Autodesk Fusion 360 part; units mm, degrees
(part 4 of 5)
sketch "Sketch4" plane through (0, 0, 22) normal (0, 0, 1) x (-1, 0, 0)
  spline S0 degree 3 poles (-268.4797, 103.3781) (-268.5106, 103.349) (-268.5781, 103.2853) (-268.6125, 103.1987) (-268.6312, 103.1517) knots 0 0 0 0 0.012573 0.027537 0.027537 0.027537 0.027537
  line L0 (-268.6312, 103.1517) -> (-268.8849, 103.183)
  spline S1 degree 3 poles (-269.284, 103.5337) (-269.2388, 103.4878) (-269.1427, 103.3903) (-269.1115, 103.2566) (-269.095, 103.1858) knots 0 0 0 0 0.01895 0.040278 0.040278 0.040278 0.040278
  line L1 (-269.095, 103.1858) -> (-269.3379, 103.1476)
  spline S2 degree 3 poles (-269.713, 103.4491) (-269.7635, 103.4479) (-269.8534, 103.4458) (-269.9303, 103.4002) (-269.9641, 103.3802) knots 0 0 0 0 0.014834 0.026419 0.026419 0.026419 0.026419
  spline S3 degree 3 poles (-269.9641, 103.3802) (-269.9879, 103.3569) (-270.0338, 103.3122) (-270.042, 103.2489) (-270.0459, 103.2185) knots 0 0 0 0 0.009682 0.0186 0.0186 0.0186 0.0186
  spline S4 degree 3 poles (-269.4572, 102.166) (-269.4912, 102.1574) (-269.5609, 102.1399) (-269.6326, 102.1378) (-269.6694, 102.1367) knots 0 0 0 0 0.010482 0.021472 0.021472 0.021472 0.021472
  spline S5 degree 3 poles (-269.6694, 102.1367) (-269.7232, 102.1382) (-269.8253, 102.1412) (-269.9227, 102.1715) (-269.9688, 102.1858) knots 0 0 0 0 0.01606 0.030471 0.030471 0.030471 0.030471
  spline S6 degree 3 poles (-252.8144, 103.5848) (-252.7657, 103.5945) (-252.6592, 103.6158) (-252.5506, 103.6174) (-252.4917, 103.6182) knots 0 0 0 0 0.014862 0.032497 0.032497 0.032497 0.032497
  line L2 (-252.4917, 103.6182) -> (-251.7291, 103.6182)
  line L3 (-251.7291, 103.6182) -> (-251.7291, 101.6182)
  line L4 (-251.7291, 101.6182) -> (-252.4794, 101.6182)
  spline S7 degree 3 poles (-252.4794, 101.6182) (-252.5489, 101.6195) (-252.6746, 101.6218) (-252.7938, 101.6613) (-252.8471, 101.6789) knots 0 0 0 0 0.020707 0.037453 0.037453 0.037453 0.037453
  spline S8 degree 3 poles (-252.8471, 101.6789) (-252.8907, 101.7018) (-252.9775, 101.7473) (-253.0353, 101.8265) (-253.064, 101.8658) knots 0 0 0 0 0.014555 0.028975 0.028975 0.028975 0.028975
  spline S9 degree 3 poles (-253.064, 101.8658) (-253.0869, 101.9079) (-253.1317, 101.9904) (-253.1389, 102.084) (-253.1425, 102.1298) knots 0 0 0 0 0.014187 0.027818 0.027818 0.027818 0.027818
  spline S10 degree 3 poles (-253.1425, 102.1298) (-253.1394, 102.1721) (-253.1334, 102.2575) (-253.0932, 102.3331) (-253.0729, 102.3713) knots 0 0 0 0 0.01257 0.025379 0.025379 0.025379 0.025379
  spline S11 degree 3 poles (-253.0729, 102.3713) (-253.0458, 102.4077) (-252.9891, 102.4838) (-252.9061, 102.53) (-252.8628, 102.5541) knots 0 0 0 0 0.013451 0.028132 0.028132 0.028132 0.028132
  spline S12 degree 3 poles (-252.8628, 102.5541) (-252.919, 102.574) (-253.0268, 102.6121) (-253.1046, 102.6956) (-253.1418, 102.7356) knots 0 0 0 0 0.017587 0.033722 0.033722 0.033722 0.033722
  spline S13 degree 3 poles (-253.1418, 102.7356) (-253.1702, 102.7808) (-253.2284, 102.8734) (-253.2356, 102.9826) (-253.2393, 103.0384) knots 0 0 0 0 0.015782 0.032266 0.032266 0.032266 0.032266
  spline S14 degree 3 poles (-253.2393, 103.0384) (-253.237, 103.0842) (-253.2323, 103.1747) (-253.1973, 103.2584) (-253.18, 103.2997) knots 0 0 0 0 0.013638 0.026971 0.026971 0.026971 0.026971
  spline S15 degree 3 poles (-253.18, 103.2997) (-253.1599, 103.3369) (-253.1218, 103.4076) (-253.0617, 103.4608) (-253.0333, 103.4859) knots 0 0 0 0 0.012583 0.02387 0.02387 0.02387 0.02387
  spline S16 degree 3 poles (-253.0333, 103.4859) (-253.0013, 103.5067) (-252.9333, 103.5507) (-252.8555, 103.573) (-252.8144, 103.5848) knots 0 0 0 0 0.011395 0.024144 0.024144 0.024144 0.024144
  spline S17 degree 3 poles (-257.0244, 103.3904) (-257.0362, 103.3956) (-257.0628, 103.4073) (-257.092, 103.4078) (-257.1083, 103.4081) knots 0 0 0 0 0.003804 0.008651 0.008651 0.008651 0.008651
  spline S18 degree 3 poles (-257.1083, 103.4081) (-257.1242, 103.4076) (-257.1603, 103.4063) (-257.196, 103.4014) (-257.2161, 103.3986) knots 0 0 0 0 0.004747 0.010826 0.010826 0.010826 0.010826
  line L5 (-257.2161, 103.3986) -> (-257.2516, 103.6155)
  spline S19 degree 3 poles (-257.2516, 103.6155) (-257.219, 103.6219) (-257.1576, 103.6338) (-257.0952, 103.6362) (-257.0661, 103.6373) knots 0 0 0 0 0.009958 0.018706 0.018706 0.018706 0.018706
  spline S20 degree 3 poles (-257.0661, 103.6373) (-257.0259, 103.6366) (-256.954, 103.6352) (-256.8879, 103.6073) (-256.8587, 103.595) knots 0 0 0 0 0.011916 0.021334 0.021334 0.021334 0.021334
  spline S21 degree 3 poles (-256.8587, 103.595) (-256.8361, 103.5802) (-256.7925, 103.5516) (-256.7672, 103.5059) (-256.755, 103.4839) knots 0 0 0 0 0.007958 0.015408 0.015408 0.015408 0.015408
  spline S22 degree 3 poles (-256.755, 103.4839) (-256.7464, 103.4484) (-256.7233, 103.3534) (-256.7243, 103.2553) (-256.725, 103.194) knots 0 0 0 0 0.010927 0.02924 0.02924 0.02924 0.02924
  line L6 (-256.725, 103.194) -> (-256.725, 102.3604)
  line L7 (-256.725, 102.3604) -> (-256.5449, 102.3604)
  line L8 (-256.5449, 102.3604) -> (-256.5449, 102.1694)
  line L9 (-256.5449, 102.1694) -> (-256.725, 102.1694)
  line L10 (-256.725, 102.1694) -> (-256.725, 101.8106)
  line L11 (-256.725, 101.8106) -> (-256.9692, 101.6633)
  line L12 (-256.9692, 101.6633) -> (-256.9692, 102.1694)
  line L13 (-256.9692, 102.1694) -> (-257.2161, 102.1694)
  line L14 (-257.2161, 102.1694) -> (-257.2161, 102.3604)
  line L15 (-257.2161, 102.3604) -> (-256.9692, 102.3604)
  line L16 (-256.9692, 102.3604) -> (-256.9692, 103.2076)
  spline S23 degree 3 poles (-256.9692, 103.2076) (-256.9688, 103.2365) (-256.9683, 103.2821) (-256.9784, 103.3265) (-256.9822, 103.3427) knots 0 0 0 0 0.008635 0.013608 0.013608 0.013608 0.013608
  spline S24 degree 3 poles (-256.9822, 103.3427) (-256.9872, 103.3522) (-256.9975, 103.3715) (-257.0154, 103.384) (-257.0244, 103.3904) knots 0 0 0 0 0.003189 0.00646 0.00646 0.00646 0.00646
  line L17 (-278.1333, 51.124) -> (-278.1333, 51.9371)
  line L18 (-278.1333, 51.9371) -> (-277.8686, 51.9371)
  line L19 (-277.8686, 51.9371) -> (-277.8686, 49.9371)
  line L20 (-277.8686, 49.9371) -> (-278.623, 49.9371)
  spline S25 degree 3 poles (-278.623, 49.9371) (-278.6817, 49.9373) (-278.7835, 49.9376) (-278.8844, 49.9507) (-278.9272, 49.9562) knots 0 0 0 0 0.017571 0.030509 0.030509 0.030509 0.030509
  spline S26 degree 3 poles (-278.9272, 49.9562) (-278.9734, 49.9656) (-279.0608, 49.9833) (-279.1378, 50.0284) (-279.1742, 50.0497) knots 0 0 0 0 0.014001 0.026564 0.026564 0.026564 0.026564
  spline S27 degree 3 poles (-279.1742, 50.0497) (-279.2061, 50.0756) (-279.2722, 50.1294) (-279.3132, 50.2041) (-279.3345, 50.2427) knots 0 0 0 0 0.012214 0.025303 0.025303 0.025303 0.025303
  spline S28 degree 3 poles (-279.3345, 50.2427) (-279.3522, 50.2856) (-279.3883, 50.373) (-279.3929, 50.4675) (-279.3952, 50.5156) knots 0 0 0 0 0.013801 0.028138 0.028138 0.028138 0.028138
  spline S29 degree 3 poles (-279.3952, 50.5156) (-279.3889, 50.5968) (-279.3765, 50.7566) (-279.2802, 50.8845) (-279.2328, 50.9474) knots 0 0 0 0 0.023898 0.046996 0.046996 0.046996 0.046996
  spline S30 degree 3 poles (-279.2328, 50.9474) (-279.1593, 50.9986) (-278.9848, 51.1201) (-278.7703, 51.1226) (-278.6462, 51.124) knots 0 0 0 0 0.026356 0.062507 0.062507 0.062507 0.062507
  line L21 (-278.6462, 51.124) -> (-278.1333, 51.124)
  line L22 (-285.0691, 51.1786) -> (-285.0691, 51.9371)
  line L23 (-285.0691, 51.9371) -> (-284.8236, 51.9371)
  line L24 (-284.8236, 51.9371) -> (-284.8236, 50.4883)
  line L25 (-284.8236, 50.4883) -> (-285.0446, 50.4883)
  line L26 (-285.0446, 50.4883) -> (-285.0446, 50.7079)
  spline S31 degree 3 poles (-285.0446, 50.7079) (-285.0692, 50.6633) (-285.1111, 50.5874) (-285.1746, 50.5288) (-285.2008, 50.5047) knots 0 0 0 0 0.015158 0.025781 0.025781 0.025781 0.025781
  spline S32 degree 3 poles (-285.2008, 50.5047) (-285.2252, 50.4904) (-285.2739, 50.4618) (-285.3303, 50.4576) (-285.3584, 50.4556) knots 0 0 0 0 0.008374 0.016702 0.016702 0.016702 0.016702
  spline S33 degree 3 poles (-285.3584, 50.4556) (-285.4009, 50.4595) (-285.4906, 50.4677) (-285.5693, 50.5116) (-285.6107, 50.5347) knots 0 0 0 0 0.012672 0.02671 0.02671 0.02671 0.02671
  line L27 (-285.6107, 50.5347) -> (-285.5262, 50.7625)
  spline S34 degree 3 poles (-285.5262, 50.7625) (-285.4968, 50.747) (-285.4403, 50.7172) (-285.3766, 50.7119) (-285.3461, 50.7093) knots 0 0 0 0 0.009849 0.018951 0.018951 0.018951 0.018951
  spline S35 degree 3 poles (-285.3461, 50.7093) (-285.3199, 50.7113) (-285.2677, 50.7154) (-285.2235, 50.7436) (-285.2015, 50.7577) knots 0 0 0 0 0.007735 0.015463 0.015463 0.015463 0.015463
  spline S36 degree 3 poles (-285.2015, 50.7577) (-285.1815, 50.7759) (-285.1403, 50.8133) (-285.1203, 50.8653) (-285.1101, 50.8921) knots 0 0 0 0 0.007973 0.016455 0.016455 0.016455 0.016455
  spline S37 degree 3 poles (-285.1101, 50.8921) (-285.0981, 50.9376) (-285.0735, 51.0315) (-285.0706, 51.1285) (-285.0691, 51.1786) knots 0 0 0 0 0.01405 0.029024 0.029024 0.029024 0.029024
  spline S38 degree 3 poles (-283.8822, 51.768) (-283.925, 51.7654) (-284.0078, 51.7606) (-284.0786, 51.7177) (-284.1128, 51.697) knots 0 0 0 0 0.012642 0.024448 0.024448 0.024448 0.024448
  spline S39 degree 3 poles (-284.1128, 51.697) (-284.1436, 51.6679) (-284.2112, 51.6042) (-284.2455, 51.5176) (-284.2642, 51.4706) knots 0 0 0 0 0.012573 0.027537 0.027537 0.027537 0.027537
  line L28 (-284.2642, 51.4706) -> (-284.518, 51.5019)
  spline S40 degree 3 poles (-284.518, 51.5019) (-284.4947, 51.5712) (-284.4495, 51.7052) (-284.3458, 51.8009) (-284.2956, 51.8471) knots 0 0 0 0 0.021523 0.041652 0.041652 0.041652 0.041652
  spline S41 degree 3 poles (-284.2956, 51.8471) (-284.2355, 51.8829) (-284.108, 51.9588) (-283.9595, 51.9661) (-283.8809, 51.9699) knots 0 0 0 0 0.020652 0.043844 0.043844 0.043844 0.043844
  spline S42 degree 3 poles (-283.8809, 51.9699) (-283.782, 51.9633) (-283.5929, 51.9508) (-283.4466, 51.8312) (-283.3768, 51.7741) knots 0 0 0 0 0.028913 0.055291 0.055291 0.055291 0.055291
  spline S43 degree 3 poles (-283.3768, 51.7741) (-283.3225, 51.6985) (-283.2054, 51.535) (-283.1957, 51.3333) (-283.1906, 51.225) knots 0 0 0 0 0.027351 0.059089 0.059089 0.059089 0.059089
  spline S44 degree 3 poles (-283.1906, 51.225) (-283.1957, 51.1131) (-283.2051, 50.9053) (-283.324, 50.7357) (-283.3788, 50.6575) knots 0 0 0 0 0.032809 0.060899 0.060899 0.060899 0.060899
  spline S45 degree 3 poles (-283.3788, 50.6575) (-283.4474, 50.5986) (-283.5878, 50.478) (-283.7726, 50.4631) (-283.8672, 50.4556) knots 0 0 0 0 0.026399 0.05408 0.05408 0.05408 0.05408
  spline S46 degree 3 poles (-283.8672, 50.4556) (-283.959, 50.4631) (-284.1388, 50.4779) (-284.2752, 50.5957) (-284.342, 50.6534) knots 0 0 0 0 0.026858 0.052633 0.052633 0.052633 0.052633
  spline S47 degree 3 poles (-284.342, 50.6534) (-284.3956, 50.7301) (-284.512, 50.8965) (-284.5212, 51.1002) (-284.5262, 51.21) knots 0 0 0 0 0.027523 0.05971 0.05971 0.05971 0.05971
  spline S48 degree 3 poles (-284.5262, 51.21) (-284.5261, 51.2191) (-284.5259, 51.2409) (-284.5252, 51.2627) (-284.5248, 51.2755) knots 0 0 0 0 0.002729 0.00655 0.00655 0.00655 0.00655
  line L29 (-284.5248, 51.2755) -> (-283.4443, 51.2755)
  spline S49 degree 3 poles (-283.4443, 51.2755) (-283.4514, 51.3482) (-283.4645, 51.4824) (-283.5433, 51.5913) (-283.5794, 51.6411) knots 0 0 0 0 0.021465 0.039604 0.039604 0.039604 0.039604
  spline S50 degree 3 poles (-283.5794, 51.6411) (-283.6226, 51.6781) (-283.7099, 51.7528) (-283.8244, 51.7629) (-283.8822, 51.768) knots 0 0 0 0 0.016633 0.033577 0.033577 0.033577 0.033577
  spline S51 degree 3 poles (-268.9524, 51.4636) (-268.9641, 51.4687) (-268.9908, 51.4805) (-269.02, 51.481) (-269.0363, 51.4813) knots 0 0 0 0 0.003804 0.008651 0.008651 0.008651 0.008651
  spline S52 degree 3 poles (-269.0363, 51.4813) (-269.0522, 51.4808) (-269.0882, 51.4795) (-269.124, 51.4745) (-269.1441, 51.4718) knots 0 0 0 0 0.004747 0.010826 0.010826 0.010826 0.010826
  line L30 (-269.1441, 51.4718) -> (-269.1796, 51.6887)
  spline S53 degree 3 poles (-269.1796, 51.6887) (-269.1469, 51.6951) (-269.0856, 51.707) (-269.0232, 51.7094) (-268.994, 51.7105) knots 0 0 0 0 0.009958 0.018706 0.018706 0.018706 0.018706
  spline S54 degree 3 poles (-268.994, 51.7105) (-268.9539, 51.7098) (-268.882, 51.7084) (-268.8159, 51.6805) (-268.7867, 51.6682) knots 0 0 0 0 0.011916 0.021334 0.021334 0.021334 0.021334
  spline S55 degree 3 poles (-268.7867, 51.6682) (-268.7641, 51.6534) (-268.7204, 51.6248) (-268.6952, 51.5791) (-268.683, 51.557) knots 0 0 0 0 0.007958 0.015408 0.015408 0.015408 0.015408
  spline S56 degree 3 poles (-268.683, 51.557) (-268.6744, 51.5215) (-268.6513, 51.4265) (-268.6523, 51.3285) (-268.653, 51.2671) knots 0 0 0 0 0.010927 0.02924 0.02924 0.02924 0.02924
  line L31 (-268.653, 51.2671) -> (-268.653, 50.4336)
  line L32 (-268.653, 50.4336) -> (-268.4729, 50.4336)
  line L33 (-268.4729, 50.4336) -> (-268.4729, 50.2426)
  line L34 (-268.4729, 50.2426) -> (-268.653, 50.2426)
  line L35 (-268.653, 50.2426) -> (-268.653, 49.8838)
  line L36 (-268.653, 49.8838) -> (-268.8972, 49.7364)
  line L37 (-268.8972, 49.7364) -> (-268.8972, 50.2426)
  line L38 (-268.8972, 50.2426) -> (-269.1441, 50.2426)
  line L39 (-269.1441, 50.2426) -> (-269.1441, 50.4336)
  line L40 (-269.1441, 50.4336) -> (-268.8972, 50.4336)
  line L41 (-268.8972, 50.4336) -> (-268.8972, 51.2808)
  spline S57 degree 3 poles (-268.8972, 51.2808) (-268.8968, 51.3097) (-268.8962, 51.3553) (-268.9064, 51.3996) (-268.9101, 51.4158) knots 0 0 0 0 0.008635 0.013608 0.013608 0.013608 0.013608
  spline S58 degree 3 poles (-268.9101, 51.4158) (-268.9152, 51.4254) (-268.9255, 51.4447) (-268.9434, 51.4572) (-268.9524, 51.4636) knots 0 0 0 0 0.003189 0.00646 0.00646 0.00646 0.00646
  spline S59 degree 3 poles (-273.7894, 51.7242) (-273.7043, 51.7218) (-273.5507, 51.7174) (-273.4181, 51.641) (-273.359, 51.6068) knots 0 0 0 0 0.025053 0.045234 0.045234 0.045234 0.045234
  spline S60 degree 3 poles (-273.359, 51.6068) (-273.3138, 51.561) (-273.2177, 51.4635) (-273.1865, 51.3298) (-273.17, 51.259) knots 0 0 0 0 0.01895 0.040278 0.040278 0.040278 0.040278
  line L42 (-273.17, 51.259) -> (-273.4129, 51.2208)
  spline S61 degree 3 poles (-273.4129, 51.2208) (-273.4218, 51.2658) (-273.4388, 51.3513) (-273.4985, 51.4146) (-273.5268, 51.4445) knots 0 0 0 0 0.013461 0.025563 0.025563 0.025563 0.025563
  spline S62 degree 3 poles (-273.5268, 51.4445) (-273.5631, 51.4671) (-273.6428, 51.5167) (-273.7369, 51.5203) (-273.788, 51.5223) knots 0 0 0 0 0.012631 0.027679 0.027679 0.027679 0.027679
  spline S63 degree 3 poles (-273.788, 51.5223) (-273.8385, 51.5211) (-273.9284, 51.519) (-274.0053, 51.4734) (-274.0391, 51.4534) knots 0 0 0 0 0.014834 0.026419 0.026419 0.026419 0.026419
  spline S64 degree 3 poles (-274.0391, 51.4534) (-274.0629, 51.4301) (-274.1088, 51.3854) (-274.117, 51.3221) (-274.1209, 51.2917) knots 0 0 0 0 0.009682 0.0186 0.0186 0.0186 0.0186
  spline S65 degree 3 poles (-274.1209, 51.2917) (-274.1178, 51.2653) (-274.1114, 51.212) (-274.0697, 51.1779) (-274.0486, 51.1607) knots 0 0 0 0 0.007652 0.015492 0.015492 0.015492 0.015492
  spline S66 degree 3 poles (-274.0486, 51.1607) (-274.0195, 51.1477) (-273.9388, 51.1114) (-273.8527, 51.0907) (-273.7976, 51.0775) knots 0 0 0 0 0.009553 0.026493 0.026493 0.026493 0.026493
  spline S67 degree 3 poles (-273.7976, 51.0775) (-273.7207, 51.0583) (-273.5935, 51.0264) (-273.4714, 50.9785) (-273.4231, 50.9595) knots 0 0 0 0 0.023737 0.039299 0.039299 0.039299 0.039299
  spline S68 degree 3 poles (-273.4231, 50.9595) (-273.3907, 50.9418) (-273.3278, 50.9074) (-273.2854, 50.8497) (-273.2648, 50.8217) knots 0 0 0 0 0.010927 0.021211 0.021211 0.021211 0.021211
  spline S69 degree 3 poles (-273.2648, 50.8217) (-273.2491, 50.7915) (-273.2174, 50.7305) (-273.2131, 50.6619) (-273.211, 50.6273) knots 0 0 0 0 0.010103 0.020373 0.020373 0.020373 0.020373
  spline S70 degree 3 poles (-273.211, 50.6273) (-273.2127, 50.5957) (-273.2163, 50.5331) (-273.2424, 50.4762) (-273.2553, 50.4479) knots 0 0 0 0 0.009394 0.018625 0.018625 0.018625 0.018625
  spline S71 degree 3 poles (-273.2553, 50.4479) (-273.2714, 50.4216) (-273.3037, 50.3688) (-273.3519, 50.3301) (-273.376, 50.3108) knots 0 0 0 0 0.009191 0.018392 0.018392 0.018392 0.018392
  spline S72 degree 3 poles (-273.376, 50.3108) (-273.3982, 50.2969) (-273.447, 50.2661) (-273.5021, 50.2487) (-273.5322, 50.2392) knots 0 0 0 0 0.007816 0.017247 0.017247 0.017247 0.017247
  spline S73 degree 3 poles (-273.5322, 50.2392) (-273.5662, 50.2306) (-273.6359, 50.2131) (-273.7076, 50.2109) (-273.7444, 50.2098) knots 0 0 0 0 0.010482 0.021472 0.021472 0.021472 0.021472
  spline S74 degree 3 poles (-273.7444, 50.2098) (-273.7982, 50.2114) (-273.9003, 50.2144) (-273.9977, 50.2446) (-274.0438, 50.259) knots 0 0 0 0 0.01606 0.030471 0.030471 0.030471 0.030471
  spline S75 degree 3 poles (-274.0438, 50.259) (-274.0831, 50.2756) (-274.1561, 50.3065) (-274.2095, 50.3649) (-274.2342, 50.392) knots 0 0 0 0 0.012607 0.023462 0.023462 0.023462 0.023462
  spline S76 degree 3 poles (-274.2342, 50.392) (-274.2533, 50.4239) (-274.2949, 50.4935) (-274.3104, 50.5733) (-274.3187, 50.6164) knots 0 0 0 0 0.011092 0.024145 0.024145 0.024145 0.024145
  line L43 (-274.3187, 50.6164) -> (-274.0786, 50.6491)
  spline S77 degree 3 poles (-274.0786, 50.6491) (-274.071, 50.6143) (-274.0563, 50.5467) (-274.0075, 50.498) (-273.9838, 50.4745) knots 0 0 0 0 0.010457 0.02025 0.02025 0.02025 0.02025
  spline S78 degree 3 poles (-273.9838, 50.4745) (-273.953, 50.4562) (-273.885, 50.4159) (-273.8056, 50.4132) (-273.7621, 50.4118) knots 0 0 0 0 0.01057 0.023371 0.023371 0.023371 0.023371
  spline S79 degree 3 poles (-273.7621, 50.4118) (-273.7127, 50.4121) (-273.6276, 50.4128) (-273.5522, 50.4515) (-273.5206, 50.4677) knots 0 0 0 0 0.014563 0.025087 0.025087 0.025087 0.025087
  spline S80 degree 3 poles (-273.5206, 50.4677) (-273.4996, 50.4863) (-273.4597, 50.5216) (-273.452, 50.574) (-273.4483, 50.5987) knots 0 0 0 0 0.00814 0.015395 0.015395 0.015395 0.015395
  spline S81 degree 3 poles (-273.4483, 50.5987) (-273.4496, 50.6142) (-273.4522, 50.6454) (-273.4696, 50.6715) (-273.4784, 50.6846) knots 0 0 0 0 0.004598 0.009239 0.009239 0.009239 0.009239
  spline S82 degree 3 poles (-273.4784, 50.6846) (-273.4906, 50.6975) (-273.5173, 50.7258) (-273.5531, 50.7415) (-273.5725, 50.7501) knots 0 0 0 0 0.005284 0.01157 0.01157 0.01157 0.01157
  spline S83 degree 3 poles (-273.5725, 50.7501) (-273.5967, 50.7577) (-273.6685, 50.7803) (-273.7412, 50.7999) (-273.7894, 50.8128) knots 0 0 0 0 0.007605 0.022583 0.022583 0.022583 0.022583
  spline S84 degree 3 poles (-273.7894, 50.8128) (-273.8636, 50.8325) (-273.9865, 50.8652) (-274.1057, 50.9093) (-274.153, 50.9268) knots 0 0 0 0 0.023005 0.038118 0.038118 0.038118 0.038118
  spline S85 degree 3 poles (-274.153, 50.9268) (-274.1852, 50.9429) (-274.2483, 50.9744) (-274.2929, 51.029) (-274.3146, 51.0557) knots 0 0 0 0 0.010681 0.020888 0.020888 0.020888 0.020888
  spline S86 degree 3 poles (-274.3146, 51.0557) (-274.3317, 51.0866) (-274.3678, 51.1518) (-274.3714, 51.2265) (-274.3733, 51.2658) knots 0 0 0 0 0.010453 0.022074 0.022074 0.022074 0.022074
  spline S87 degree 3 poles (-274.3733, 51.2658) (-274.3701, 51.3064) (-274.3637, 51.3888) (-274.3226, 51.4606) (-274.3017, 51.497) knots 0 0 0 0 0.012054 0.024479 0.024479 0.024479 0.024479
  spline S88 degree 3 poles (-274.3017, 51.497) (-274.2745, 51.5314) (-274.2181, 51.6027) (-274.1369, 51.6436) (-274.095, 51.6648) knots 0 0 0 0 0.013001 0.026908 0.026908 0.026908 0.026908
  spline S89 degree 3 poles (-274.095, 51.6648) (-274.0475, 51.6821) (-273.9489, 51.7181) (-273.8439, 51.7221) (-273.7894, 51.7242) knots 0 0 0 0 0.015065 0.0313 0.0313 0.0313 0.0313
  line L44 (-272.8835, 50.2426) -> (-272.8835, 51.6914)
  line L45 (-272.8835, 51.6914) -> (-272.6639, 51.6914)
  line L46 (-272.6639, 51.6914) -> (-272.6639, 51.4786)
  spline S90 degree 3 poles (-272.6639, 51.4786) (-272.6028, 51.5502) (-272.4816, 51.6924) (-272.2962, 51.7136) (-272.2041, 51.7242) knots 0 0 0 0 0.027153 0.053891 0.053891 0.053891 0.053891
  spline S91 degree 3 poles (-272.2041, 51.7242) (-272.1624, 51.7222) (-272.08, 51.7184) (-272.0028, 51.6894) (-271.9647, 51.6751) knots 0 0 0 0 0.012458 0.024577 0.024577 0.024577 0.024577
  spline S92 degree 3 poles (-271.9647, 51.6751) (-271.9308, 51.6587) (-271.8677, 51.6281) (-271.8212, 51.5758) (-271.7996, 51.5516) knots 0 0 0 0 0.01116 0.020794 0.020794 0.020794 0.020794
  spline S93 degree 3 poles (-271.7996, 51.5516) (-271.7829, 51.5246) (-271.7477, 51.4681) (-271.7321, 51.4034) (-271.7239, 51.3695) knots 0 0 0 0 0.009458 0.019838 0.019838 0.019838 0.019838
  spline S94 degree 3 poles (-271.7239, 51.3695) (-271.7196, 51.3384) (-271.709, 51.2624) (-271.7089, 51.1856) (-271.7089, 51.1403) knots 0 0 0 0 0.009413 0.022992 0.022992 0.022992 0.022992
  line L47 (-271.7089, 51.1403) -> (-271.7089, 50.2426)
  line L48 (-271.7089, 50.2426) -> (-271.9545, 50.2426)
  line L49 (-271.9545, 50.2426) -> (-271.9545, 51.0461)
  spline S95 degree 3 poles (-271.9545, 51.0461) (-271.9542, 51.0999) (-271.9538, 51.1867) (-271.9652, 51.2726) (-271.9695, 51.3053) knots 0 0 0 0 0.016103 0.02599 0.02599 0.02599 0.02599
  spline S96 degree 3 poles (-271.9695, 51.3053) (-271.9791, 51.3357) (-271.9981, 51.3954) (-272.0448, 51.437) (-272.0677, 51.4575) knots 0 0 0 0 0.009371 0.018407 0.018407 0.018407 0.018407
  spline S97 degree 3 poles (-272.0677, 51.4575) (-272.095, 51.4736) (-272.1521, 51.5073) (-272.2185, 51.5109) (-272.2533, 51.5127) knots 0 0 0 0 0.009358 0.019615 0.019615 0.019615 0.019615
  spline S98 degree 3 poles (-272.2533, 51.5127) (-272.2896, 51.5103) (-272.3625, 51.5055) (-272.4278, 51.4726) (-272.4606, 51.4561) knots 0 0 0 0 0.010803 0.021692 0.021692 0.021692 0.021692
  spline S99 degree 3 poles (-272.4606, 51.4561) (-272.4904, 51.4358) (-272.5491, 51.3959) (-272.5817, 51.3329) (-272.5977, 51.3019) knots 0 0 0 0 0.010635 0.020922 0.020922 0.020922 0.020922
  spline S100 degree 3 poles (-272.5977, 51.3019) (-272.6094, 51.2623) (-272.6366, 51.1701) (-272.6375, 51.0738) (-272.638, 51.0188) knots 0 0 0 0 0.012329 0.028714 0.028714 0.028714 0.028714
  line L50 (-272.638, 51.0188) -> (-272.638, 50.2426)
  line L51 (-272.638, 50.2426) -> (-272.8835, 50.2426)
  spline S101 degree 3 poles (-271.2826, 51.4636) (-271.2943, 51.4687) (-271.3209, 51.4805) (-271.3501, 51.481) (-271.3665, 51.4813) knots 0 0 0 0 0.003804 0.008651 0.008651 0.008651 0.008651
  spline S102 degree 3 poles (-271.3665, 51.4813) (-271.3823, 51.4808) (-271.4184, 51.4795) (-271.4542, 51.4745) (-271.4743, 51.4718) knots 0 0 0 0 0.004747 0.010826 0.010826 0.010826 0.010826
  line L52 (-271.4743, 51.4718) -> (-271.5097, 51.6887)
  spline S103 degree 3 poles (-269.9688, 102.1858) (-270.0081, 102.2024) (-270.0811, 102.2333) (-270.1345, 102.2918) (-270.1591, 102.3188) knots 0 0 0 0 0.012608 0.023462 0.023462 0.023462 0.023462
  spline S104 degree 3 poles (-270.1591, 102.3188) (-270.1783, 102.3508) (-270.2199, 102.4204) (-270.2354, 102.5001) (-270.2437, 102.5432) knots 0 0 0 0 0.011092 0.024145 0.024145 0.024145 0.024145
  spline S105 degree 3 poles (-270.0036, 102.5759) (-269.996, 102.5411) (-269.9813, 102.4735) (-269.9324, 102.4249) (-269.9088, 102.4013) knots 0 0 0 0 0.010457 0.02025 0.02025 0.02025 0.02025
  spline S106 degree 3 poles (-270.02, 103.5916) (-269.9725, 103.6089) (-269.8738, 103.6449) (-269.7688, 103.6489) (-269.7144, 103.651) knots 0 0 0 0 0.015065 0.0313 0.0313 0.0313 0.0313
  spline S107 degree 3 poles (-269.7144, 103.651) (-269.6293, 103.6486) (-269.4757, 103.6442) (-269.3431, 103.5678) (-269.284, 103.5337) knots 0 0 0 0 0.025053 0.045234 0.045234 0.045234 0.045234
  spline S108 degree 3 poles (-270.3788, 51.6914) (-270.3671, 51.6641) (-270.3426, 51.6068) (-270.3341, 51.5451) (-270.3297, 51.5127) knots 0 0 0 0 0.008862 0.018609 0.018609 0.018609 0.018609
  spline S109 degree 3 poles (-270.3297, 51.5127) (-270.2864, 51.5478) (-270.2056, 51.6134) (-270.1109, 51.6564) (-270.067, 51.6764) knots 0 0 0 0 0.016644 0.031058 0.031058 0.031058 0.031058
  spline S110 degree 3 poles (-270.067, 51.6764) (-270.0238, 51.6903) (-269.9357, 51.7187) (-269.8433, 51.7223) (-269.7962, 51.7242) knots 0 0 0 0 0.013561 0.027613 0.027613 0.027613 0.027613
  spline S111 degree 3 poles (-269.7962, 51.7242) (-269.7236, 51.7213) (-269.59, 51.7159) (-269.4796, 51.6415) (-269.4292, 51.6075) knots 0 0 0 0 0.021312 0.039186 0.039186 0.039186 0.039186
  spline S112 degree 3 poles (-269.4292, 51.6075) (-269.3918, 51.5656) (-269.3161, 51.4805) (-269.3061, 51.367) (-269.301, 51.3094) knots 0 0 0 0 0.016401 0.033233 0.033233 0.033233 0.033233
  spline S113 degree 3 poles (-268.8849, 103.183) (-268.8616, 103.2523) (-268.8165, 103.3862) (-268.7127, 103.4819) (-268.6626, 103.5282) knots 0 0 0 0 0.021523 0.041652 0.041652 0.041652 0.041652
  spline S114 degree 3 poles (-268.6626, 103.5282) (-268.6025, 103.564) (-268.475, 103.6399) (-268.3264, 103.6472) (-268.2478, 103.651) knots 0 0 0 0 0.020652 0.043844 0.043844 0.043844 0.043844
  spline S115 degree 3 poles (-268.2478, 103.651) (-268.1489, 103.6444) (-267.9598, 103.6319) (-267.8135, 103.5123) (-267.7437, 103.4552) knots 0 0 0 0 0.028913 0.055291 0.055291 0.055291 0.055291
  spline S116 degree 3 poles (-267.7437, 103.4552) (-267.6895, 103.3795) (-267.5723, 103.2161) (-267.5627, 103.0144) (-267.5575, 102.9061) knots 0 0 0 0 0.027351 0.059089 0.059089 0.059089 0.059089
  spline S117 degree 3 poles (-267.5575, 102.9061) (-267.5626, 102.7942) (-267.5721, 102.5864) (-267.6909, 102.4168) (-267.7458, 102.3386) knots 0 0 0 0 0.032809 0.060899 0.060899 0.060899 0.060899
  spline S118 degree 3 poles (-267.7458, 102.3386) (-267.8143, 102.2797) (-267.9548, 102.1591) (-268.1396, 102.1442) (-268.2342, 102.1367) knots 0 0 0 0 0.026399 0.05408 0.05408 0.05408 0.05408
  spline S119 degree 3 poles (-268.2342, 102.1367) (-268.3259, 102.1442) (-268.5058, 102.159) (-268.6422, 102.2768) (-268.7089, 102.3345) knots 0 0 0 0 0.026858 0.052633 0.052633 0.052633 0.052633
  spline S120 degree 3 poles (-268.7089, 102.3345) (-268.7626, 102.4112) (-268.8789, 102.5776) (-268.8881, 102.7813) (-268.8931, 102.8911) knots 0 0 0 0 0.027523 0.05971 0.05971 0.05971 0.05971
  spline S121 degree 3 poles (-268.8931, 102.8911) (-268.893, 102.9002) (-268.8928, 102.922) (-268.8921, 102.9438) (-268.8917, 102.9566) knots 0 0 0 0 0.002729 0.00655 0.00655 0.00655 0.00655
  spline S122 degree 3 poles (-267.9463, 103.3222) (-267.9896, 103.3592) (-268.0769, 103.4339) (-268.1914, 103.444) (-268.2492, 103.4491) knots 0 0 0 0 0.016633 0.033577 0.033577 0.033577 0.033577
  spline S123 degree 3 poles (-268.2492, 103.4491) (-268.292, 103.4465) (-268.3747, 103.4416) (-268.4455, 103.3988) (-268.4797, 103.3781) knots 0 0 0 0 0.012642 0.024448 0.024448 0.024448 0.024448
  spline S124 degree 3 poles (-269.668, 50.261) (-269.7187, 50.2461) (-269.826, 50.2145) (-269.9378, 50.2115) (-269.9968, 50.2098) knots 0 0 0 0 0.015787 0.033398 0.033398 0.033398 0.033398
  spline S125 degree 3 poles (-269.9968, 50.2098) (-270.0532, 50.2108) (-270.1557, 50.2125) (-270.2541, 50.2408) (-270.2983, 50.2535) knots 0 0 0 0 0.01685 0.030582 0.030582 0.030582 0.030582
  spline S126 degree 3 poles (-270.2983, 50.2535) (-270.3333, 50.2677) (-270.3971, 50.2937) (-270.4465, 50.3416) (-270.4688, 50.3633) knots 0 0 0 0 0.011204 0.020452 0.020452 0.020452 0.020452
  spline S127 degree 3 poles (-270.4688, 50.3633) (-270.4858, 50.3876) (-270.5215, 50.4385) (-270.537, 50.4988) (-270.5452, 50.5304) knots 0 0 0 0 0.008807 0.018509 0.018509 0.018509 0.018509
  spline S128 degree 3 poles (-270.5452, 50.5304) (-270.5487, 50.5597) (-270.5578, 50.6349) (-270.5576, 50.7107) (-270.5575, 50.7569) knots 0 0 0 0 0.008848 0.022698 0.022698 0.022698 0.022698
  line L53 (-270.5575, 50.7569) -> (-270.5575, 51.0843)
  spline S129 degree 3 poles (-270.5575, 51.0843) (-270.5569, 51.1776) (-270.556, 51.3222) (-270.5687, 51.4663) (-270.5732, 51.5175) knots 0 0 0 0 0.027953 0.043363 0.043363 0.043363 0.043363
  spline S130 degree 3 poles (-269.3379, 103.1476) (-269.3468, 103.1926) (-269.3638, 103.2781) (-269.4235, 103.3414) (-269.4518, 103.3713) knots 0 0 0 0 0.013461 0.025563 0.025563 0.025563 0.025563
  spline S131 degree 3 poles (-267.0834, 51.6464) (-267.0258, 51.6171) (-266.912, 51.5591) (-266.834, 51.4582) (-266.7955, 51.4083) knots 0 0 0 0 0.019136 0.037772 0.037772 0.037772 0.037772
  spline S132 degree 3 poles (-266.7955, 51.4083) (-266.7649, 51.3532) (-266.7026, 51.2412) (-266.6914, 51.1136) (-266.6857, 51.0489) knots 0 0 0 0 0.018713 0.037965 0.037965 0.037965 0.037965
  line L54 (-266.6857, 51.0489) -> (-266.9354, 51.027)
  spline S133 degree 3 poles (-266.9354, 51.027) (-266.9424, 51.0735) (-266.9556, 51.1605) (-266.9981, 51.2375) (-267.0179, 51.2733) knots 0 0 0 0 0.013975 0.026155 0.026155 0.026155 0.026155
  spline S134 degree 3 poles (-267.0179, 51.2733) (-267.0438, 51.3044) (-267.0993, 51.3709) (-267.1775, 51.4087) (-267.2191, 51.4288) knots 0 0 0 0 0.012002 0.025694 0.025694 0.025694 0.025694
  spline S135 degree 3 poles (-267.2191, 51.4288) (-267.267, 51.4461) (-267.3661, 51.482) (-267.4715, 51.486) (-267.5261, 51.4881) knots 0 0 0 0 0.015163 0.031432 0.031432 0.031432 0.031432
  spline S136 degree 3 poles (-267.5261, 51.4881) (-267.574, 51.4867) (-267.6653, 51.4839) (-267.7522, 51.4563) (-267.7935, 51.4431) knots 0 0 0 0 0.014301 0.027232 0.027232 0.027232 0.027232
  spline S137 degree 3 poles (-267.7935, 51.4431) (-267.8289, 51.4277) (-267.8954, 51.3988) (-267.9436, 51.3448) (-267.9661, 51.3197) knots 0 0 0 0 0.011435 0.021444 0.021444 0.021444 0.021444
  spline S138 degree 3 poles (-267.9661, 51.3197) (-267.9826, 51.2931) (-268.0152, 51.2406) (-268.0202, 51.1789) (-268.0227, 51.1484) knots 0 0 0 0 0.009237 0.018267 0.018267 0.018267 0.018267
  spline S139 degree 3 poles (-268.0227, 51.1484) (-268.0206, 51.1183) (-268.0164, 51.0588) (-267.984, 51.0087) (-267.9681, 50.9841) knots 0 0 0 0 0.008921 0.017573 0.017573 0.017573 0.017573
  spline S140 degree 3 poles (-267.9681, 50.9841) (-267.9451, 50.9609) (-267.8935, 50.909) (-267.8256, 50.8814) (-267.788, 50.866) knots 0 0 0 0 0.009698 0.021725 0.021725 0.021725 0.021725
  spline S141 degree 3 poles (-267.788, 50.866) (-267.7451, 50.8523) (-267.6278, 50.8147) (-267.5079, 50.7864) (-267.432, 50.7685) knots 0 0 0 0 0.013533 0.036931 0.036931 0.036931 0.036931
  spline S142 degree 3 poles (-267.432, 50.7685) (-267.353, 50.7496) (-267.2209, 50.7181) (-267.0961, 50.665) (-267.0459, 50.6437) knots 0 0 0 0 0.024297 0.040637 0.040637 0.040637 0.040637
  spline S143 degree 3 poles (-267.0459, 50.6437) (-267.0019, 50.6183) (-266.9185, 50.5701) (-266.86, 50.4936) (-266.8324, 50.4575) knots 0 0 0 0 0.015064 0.02858 0.02858 0.02858 0.02858
  spline S144 degree 3 poles (-266.8324, 50.4575) (-266.8119, 50.419) (-266.7704, 50.3411) (-266.7649, 50.2531) (-266.7621, 50.2085) knots 0 0 0 0 0.012908 0.026139 0.026139 0.026139 0.026139
  spline S145 degree 3 poles (-266.7621, 50.2085) (-266.7658, 50.1586) (-266.7734, 50.0579) (-266.823, 49.9698) (-266.8481, 49.9254) knots 0 0 0 0 0.014805 0.02991 0.02991 0.02991 0.02991
  spline S146 degree 3 poles (-266.8481, 49.9254) (-266.8809, 49.8838) (-266.9489, 49.7977) (-267.0479, 49.7501) (-267.0991, 49.7255) knots 0 0 0 0 0.01568 0.032466 0.032466 0.032466 0.032466
  spline S147 degree 3 poles (-267.0991, 49.7255) (-267.1566, 49.7056) (-267.2755, 49.6646) (-267.4012, 49.6598) (-267.4661, 49.6573) knots 0 0 0 0 0.018164 0.037509 0.037509 0.037509 0.037509
  spline S148 degree 3 poles (-267.4661, 49.6573) (-267.5365, 49.6597) (-267.6709, 49.6642) (-267.7979, 49.7081) (-267.8583, 49.7289) knots 0 0 0 0 0.021001 0.040071 0.040071 0.040071 0.040071
  spline S149 degree 3 poles (-267.8583, 49.7289) (-267.9112, 49.755) (-268.0142, 49.8056) (-268.0851, 49.8958) (-268.1196, 49.9397) knots 0 0 0 0 0.017437 0.033952 0.033952 0.033952 0.033952
  spline S150 degree 3 poles (-268.1196, 49.9397) (-268.1465, 49.9881) (-268.2012, 50.0862) (-268.2122, 50.1981) (-268.2178, 50.2549) knots 0 0 0 0 0.016416 0.033327 0.033327 0.033327 0.033327
  line L55 (-268.2178, 50.2549) -> (-267.964, 50.274)
  spline S151 degree 3 poles (-267.964, 50.274) (-267.9545, 50.2158) (-267.9365, 50.1062) (-267.861, 50.0254) (-267.8256, 49.9875) knots 0 0 0 0 0.017238 0.032462 0.032462 0.032462 0.032462
  spline S152 degree 3 poles (-267.8256, 49.9875) (-267.778, 49.9593) (-267.6711, 49.896) (-267.5463, 49.8925) (-267.477, 49.8906) knots 0 0 0 0 0.016321 0.036707 0.036707 0.036707 0.036707
  spline S153 degree 3 poles (-267.477, 49.8906) (-267.4061, 49.8917) (-267.2818, 49.8936) (-267.1735, 49.9531) (-267.1271, 49.9786) knots 0 0 0 0 0.02087 0.036564 0.036564 0.036564 0.036564
  spline S154 degree 3 poles (-267.1271, 49.9786) (-267.095, 50.0086) (-267.0332, 50.0666) (-267.0224, 50.1504) (-267.0172, 50.1907) knots 0 0 0 0 0.012728 0.024562 0.024562 0.024562 0.024562
  spline S155 degree 3 poles (-267.0172, 50.1907) (-267.0204, 50.225) (-267.0265, 50.2928) (-267.0723, 50.3431) (-267.095, 50.3681) knots 0 0 0 0 0.010013 0.019843 0.019843 0.019843 0.019843
  spline S156 degree 3 poles (-267.095, 50.3681) (-267.1403, 50.3933) (-267.2648, 50.4627) (-267.4049, 50.492) (-267.494, 50.5107) knots 0 0 0 0 0.01549 0.042576 0.042576 0.042576 0.042576
  spline S157 degree 3 poles (-267.494, 50.5107) (-267.5854, 50.5311) (-267.7357, 50.5646) (-267.8801, 50.6175) (-267.9367, 50.6382) knots 0 0 0 0 0.028046 0.046113 0.046113 0.046113 0.046113
  spline S158 degree 3 poles (-267.9367, 50.6382) (-267.99, 50.6653) (-268.0899, 50.716) (-268.1613, 50.802) (-268.1946, 50.8422) knots 0 0 0 0 0.017708 0.033187 0.033187 0.033187 0.033187
  spline S159 degree 3 poles (-268.1946, 50.8422) (-268.2189, 50.8854) (-268.2684, 50.9738) (-268.2746, 51.075) (-268.2778, 51.1266) knots 0 0 0 0 0.014678 0.02998 0.02998 0.02998 0.02998
  spline S160 degree 3 poles (-268.2778, 51.1266) (-268.2738, 51.1794) (-268.2656, 51.2864) (-268.2131, 51.38) (-268.1864, 51.4274) knots 0 0 0 0 0.015669 0.031781 0.031781 0.031781 0.031781
  spline S161 degree 3 poles (-268.1864, 51.4274) (-268.1518, 51.4723) (-268.0804, 51.5647) (-267.977, 51.6191) (-267.9238, 51.6471) knots 0 0 0 0 0.016779 0.034595 0.034595 0.034595 0.034595
  spline S162 degree 3 poles (-267.9238, 51.6471) (-267.8638, 51.67) (-267.7397, 51.7173) (-267.607, 51.7227) (-267.5384, 51.7255) knots 0 0 0 0 0.019123 0.039562 0.039562 0.039562 0.039562
  spline S163 degree 3 poles (-267.5384, 51.7255) (-267.4544, 51.7234) (-267.2987, 51.7194) (-267.1513, 51.6694) (-267.0834, 51.6464) knots 0 0 0 0 0.025027 0.046416 0.046416 0.046416 0.046416
  line L56 (-282.0719, 50.8225) -> (-281.7785, 51.9371)
  line L57 (-281.7785, 51.9371) -> (-281.5221, 51.9371)
  line L58 (-281.5221, 51.9371) -> (-281.0787, 50.4883)
  line L59 (-281.0787, 50.4883) -> (-281.3324, 50.4883)
  line L60 (-281.3324, 50.4883) -> (-281.563, 51.3246)
  line L61 (-281.563, 51.3246) -> (-281.6489, 51.6356)
  spline S164 degree 3 poles (-281.6489, 51.6356) (-281.6561, 51.6069) (-281.6809, 51.5072) (-281.7061, 51.4077) (-281.724, 51.3369) knots 0 0 0 0 0.008892 0.030805 0.030805 0.030805 0.030805
  line L62 (-281.724, 51.3369) -> (-281.9545, 50.4883)
  line L63 (-281.9545, 50.4883) -> (-282.2069, 50.4883)
  line L64 (-282.2069, 50.4883) -> (-282.4238, 51.3287)
  line L65 (-282.4238, 51.3287) -> (-282.4961, 51.6056)
  line L66 (-282.4961, 51.6056) -> (-282.5794, 51.326)
  line L67 (-282.5794, 51.326) -> (-282.8277, 50.4883)
  line L68 (-282.8277, 50.4883) -> (-283.0664, 50.4883)
  line L69 (-283.0664, 50.4883) -> (-282.6135, 51.9371)
  line L70 (-282.6135, 51.9371) -> (-282.3584, 51.9371)
  line L71 (-282.3584, 51.9371) -> (-282.1278, 51.0695)
  line L72 (-282.1278, 51.0695) -> (-282.0719, 50.8225)
  spline S165 degree 3 poles (-280.2888, 51.9699) (-280.1933, 51.9629) (-280.0086, 51.9493) (-279.8659, 51.8317) (-279.797, 51.7748) knots 0 0 0 0 0.027936 0.054087 0.054087 0.054087 0.054087
  spline S166 degree 3 poles (-279.797, 51.7748) (-279.7424, 51.6982) (-279.6231, 51.5308) (-279.6142, 51.3245) (-279.6094, 51.2127) knots 0 0 0 0 0.027653 0.060391 0.060391 0.060391 0.060391
  spline S167 degree 3 poles (-279.6094, 51.2127) (-279.615, 51.0908) (-279.6253, 50.8665) (-279.768, 50.6949) (-279.8331, 50.6165) knots 0 0 0 0 0.035471 0.065242 0.065242 0.065242 0.065242
  spline S168 degree 3 poles (-279.8331, 50.6165) (-279.8998, 50.5696) (-280.0365, 50.4734) (-280.2034, 50.4616) (-280.2888, 50.4556) knots 0 0 0 0 0.023996 0.049149 0.049149 0.049149 0.049149
  spline S169 degree 3 poles (-280.2888, 50.4556) (-280.383, 50.4628) (-280.5665, 50.477) (-280.7082, 50.5942) (-280.7772, 50.6513) knots 0 0 0 0 0.027586 0.05378 0.05378 0.05378 0.05378
  spline S170 degree 3 poles (-280.7772, 50.6513) (-280.8324, 50.7262) (-280.9507, 50.8864) (-280.9612, 51.0859) (-280.9668, 51.1923) knots 0 0 0 0 0.027308 0.058452 0.058452 0.058452 0.058452
  spline S171 degree 3 poles (-280.9668, 51.1923) (-280.9652, 51.2766) (-280.9622, 51.4284) (-280.9073, 51.5696) (-280.8829, 51.6322) knots 0 0 0 0 0.025071 0.045099 0.045099 0.045099 0.045099
  spline S172 degree 3 poles (-280.8829, 51.6322) (-280.8517, 51.6827) (-280.789, 51.7841) (-280.6889, 51.8488) (-280.6387, 51.8812) knots 0 0 0 0 0.017574 0.035265 0.035265 0.035265 0.035265
  spline S173 degree 3 poles (-280.6387, 51.8812) (-280.5838, 51.9071) (-280.4729, 51.9593) (-280.3505, 51.9663) (-280.2888, 51.9699) knots 0 0 0 0 0.018034 0.036399 0.036399 0.036399 0.036399
  spline S174 degree 3 poles (-255.7141, 103.651) (-255.6186, 103.644) (-255.4339, 103.6304) (-255.2912, 103.5128) (-255.2223, 103.4559) knots 0 0 0 0 0.027936 0.054087 0.054087 0.054087 0.054087
  spline S175 degree 3 poles (-255.2223, 103.4559) (-255.1677, 103.3793) (-255.0484, 103.2119) (-255.0395, 103.0056) (-255.0347, 102.8938) knots 0 0 0 0 0.027653 0.060391 0.060391 0.060391 0.060391
  spline S176 degree 3 poles (-255.0347, 102.8938) (-255.0403, 102.7719) (-255.0506, 102.5476) (-255.1933, 102.3759) (-255.2584, 102.2976) knots 0 0 0 0 0.035471 0.065242 0.065242 0.065242 0.065242
  spline S177 degree 3 poles (-255.2584, 102.2976) (-255.3251, 102.2507) (-255.4618, 102.1545) (-255.6287, 102.1427) (-255.7141, 102.1367) knots 0 0 0 0 0.023996 0.049149 0.049149 0.049149 0.049149
  spline S178 degree 3 poles (-255.7141, 102.1367) (-255.8083, 102.1439) (-255.9918, 102.1581) (-256.1335, 102.2753) (-256.2025, 102.3324) knots 0 0 0 0 0.027586 0.05378 0.05378 0.05378 0.05378
  spline S179 degree 3 poles (-256.2025, 102.3324) (-256.2577, 102.4073) (-256.376, 102.5675) (-256.3865, 102.767) (-256.3921, 102.8734) knots 0 0 0 0 0.027308 0.058452 0.058452 0.058452 0.058452
  spline S180 degree 3 poles (-256.3921, 102.8734) (-256.3905, 102.9577) (-256.3875, 103.1095) (-256.3326, 103.2506) (-256.3082, 103.3133) knots 0 0 0 0 0.025071 0.045099 0.045099 0.045099 0.045099
  spline S181 degree 3 poles (-256.3082, 103.3133) (-256.277, 103.3638) (-256.2143, 103.4652) (-256.1142, 103.5298) (-256.064, 103.5623) knots 0 0 0 0 0.017574 0.035265 0.035265 0.035265 0.035265
  spline S182 degree 3 poles (-256.064, 103.5623) (-256.0091, 103.5882) (-255.8982, 103.6404) (-255.7758, 103.6474) (-255.7141, 103.651) knots 0 0 0 0 0.018034 0.036399 0.036399 0.036399 0.036399
  spline S183 degree 3 poles (-254.1602, 103.651) (-254.0648, 103.644) (-253.88, 103.6304) (-253.7373, 103.5128) (-253.6684, 103.4559) knots 0 0 0 0 0.027936 0.054087 0.054087 0.054087 0.054087
  spline S184 degree 3 poles (-253.6684, 103.4559) (-253.6138, 103.3793) (-253.4945, 103.2119) (-253.4856, 103.0056) (-253.4808, 102.8938) knots 0 0 0 0 0.027653 0.060391 0.060391 0.060391 0.060391
  spline S185 degree 3 poles (-253.4808, 102.8938) (-253.4864, 102.7719) (-253.4967, 102.5476) (-253.6394, 102.3759) (-253.7045, 102.2976) knots 0 0 0 0 0.035471 0.065242 0.065242 0.065242 0.065242
  spline S186 degree 3 poles (-253.7045, 102.2976) (-253.7713, 102.2507) (-253.9079, 102.1545) (-254.0748, 102.1427) (-254.1602, 102.1367) knots 0 0 0 0 0.023996 0.049149 0.049149 0.049149 0.049149
  spline S187 degree 3 poles (-254.1602, 102.1367) (-254.2544, 102.1439) (-254.438, 102.1581) (-254.5796, 102.2753) (-254.6486, 102.3324) knots 0 0 0 0 0.027586 0.05378 0.05378 0.05378 0.05378
  spline S188 degree 3 poles (-254.6486, 102.3324) (-254.7038, 102.4073) (-254.8221, 102.5675) (-254.8326, 102.767) (-254.8382, 102.8734) knots 0 0 0 0 0.027308 0.058452 0.058452 0.058452 0.058452
  spline S189 degree 3 poles (-254.8382, 102.8734) (-254.8366, 102.9577) (-254.8336, 103.1095) (-254.7787, 103.2506) (-254.7543, 103.3133) knots 0 0 0 0 0.025071 0.045099 0.045099 0.045099 0.045099
  spline S190 degree 3 poles (-254.7543, 103.3133) (-254.7231, 103.3638) (-254.6604, 103.4652) (-254.5603, 103.5298) (-254.5101, 103.5623) knots 0 0 0 0 0.017574 0.035265 0.035265 0.035265 0.035265
  spline S191 degree 3 poles (-254.5101, 103.5623) (-254.4552, 103.5882) (-254.3443, 103.6404) (-254.2219, 103.6474) (-254.1602, 103.651) knots 0 0 0 0 0.018034 0.036399 0.036399 0.036399 0.036399
  spline S192 degree 3 poles (-271.4306, 103.3781) (-271.4615, 103.349) (-271.529, 103.2853) (-271.5634, 103.1987) (-271.5821, 103.1517) knots 0 0 0 0 0.012573 0.027537 0.027537 0.027537 0.027537
  line L73 (-271.5821, 103.1517) -> (-271.8358, 103.183)
  spline S193 degree 3 poles (-271.8358, 103.183) (-271.8125, 103.2523) (-271.7674, 103.3862) (-271.6636, 103.4819) (-271.6134, 103.5282) knots 0 0 0 0 0.021523 0.041652 0.041652 0.041652 0.041652
  spline S194 degree 3 poles (-272.5725, 103.4081) (-272.5883, 103.4076) (-272.6244, 103.4063) (-272.6602, 103.4014) (-272.6803, 103.3986) knots 0 0 0 0 0.004747 0.010826 0.010826 0.010826 0.010826
  line L74 (-272.6803, 103.3986) -> (-272.7158, 103.6155)
  line L75 (-265.9218, 103.6182) -> (-265.6571, 103.6182)
  line L76 (-265.6571, 103.6182) -> (-265.6571, 101.6182)
  spline S195 degree 3 poles (-266.9504, 101.6721) (-266.9947, 101.6939) (-267.085, 101.7384) (-267.1432, 101.8206) (-267.1728, 101.8624) knots 0 0 0 0 0.014568 0.029686 0.029686 0.029686 0.029686
  spline S196 degree 3 poles (-267.1728, 101.8624) (-267.1971, 101.9093) (-267.246, 102.004) (-267.2527, 102.1103) (-267.256, 102.1639) knots 0 0 0 0 0.015657 0.031584 0.031584 0.031584 0.031584
  line L77 (-259.9009, 59) -> (-249.9009, 59)
  line L78 (-249.9009, 59) -> (-249.9009, 53)
  line L79 (-249.9009, 53) -> (-259.9009, 53)
  line L80 (-259.9009, 53) -> (-259.9009, 59)
  arc A0 (-260.2748, 92.3293) -> (-257.2248, 89.2793) centre (-257.2248, 92.3293) ccw
  line L81 (-260.2748, 92.3293) -> (-260.2748, 97.7293)
  arc A1 (-257.2248, 100.7793) -> (-260.2748, 97.7293) centre (-257.2248, 97.7293) ccw
  line L82 (-257.2248, 100.7793) -> (-251.8248, 100.7793)
  arc A2 (-248.7748, 97.7293) -> (-251.8248, 100.7793) centre (-251.8248, 97.7293) ccw
  line L83 (-248.7748, 97.7293) -> (-248.7748, 92.3293)
  arc A3 (-251.8248, 89.2793) -> (-248.7748, 92.3293) centre (-251.8248, 92.3293) ccw
  line L84 (-251.8248, 89.2793) -> (-257.2248, 89.2793)
  line L85 (-263.1698, 97.5713) -> (-263.1698, 92.1713)
  arc A4 (-266.2198, 89.1213) -> (-263.1698, 92.1713) centre (-266.2198, 92.1713) ccw
  line L86 (-266.2198, 89.1213) -> (-271.6198, 89.1213)
  arc A5 (-274.6698, 92.1713) -> (-271.6198, 89.1213) centre (-271.6198, 92.1713) ccw
  line L87 (-274.6698, 92.1713) -> (-274.6698, 97.5713)
  arc A6 (-271.6198, 100.6213) -> (-274.6698, 97.5713) centre (-271.6198, 97.5713) ccw
  line L88 (-271.6198, 100.6213) -> (-266.2198, 100.6213)
  arc A7 (-263.1698, 97.5713) -> (-266.2198, 100.6213) centre (-266.2198, 97.5713) ccw
  circle A8 centre (-270.3911, 55.7056) radius 3
  circle A9 centre (-281.5411, 55.7956) radius 3
  line L89 (-248.7148, 86.5518) -> (-247.9448, 86.5518)
  arc A10 (-247.6948, 86.5414) -> (-247.9448, 86.5518) centre (-247.9448, 83.5518) ccw
  arc A11 (-247.4448, 86.5518) -> (-247.6948, 86.5414) centre (-247.4448, 83.5518) ccw
  line L90 (-247.4448, 86.5518) -> (-246.6748, 86.5518)
  arc A12 (-246.4248, 86.5414) -> (-246.6748, 86.5518) centre (-246.6748, 83.5518) ccw
  arc A13 (-246.1748, 86.5518) -> (-246.4248, 86.5414) centre (-246.1748, 83.5518) ccw
  line L91 (-246.1748, 86.5518) -> (-245.4048, 86.5518)
  arc A14 (-245.1548, 86.5414) -> (-245.4048, 86.5518) centre (-245.4048, 83.5518) ccw
  arc A15 (-244.9048, 86.5518) -> (-245.1548, 86.5414) centre (-244.9048, 83.5518) ccw
  line L92 (-244.9048, 86.5518) -> (-244.1348, 86.5518)
  arc A16 (-243.8848, 86.5414) -> (-244.1348, 86.5518) centre (-244.1348, 83.5518) ccw
  arc A17 (-243.6348, 86.5518) -> (-243.8848, 86.5414) centre (-243.6348, 83.5518) ccw
  line L93 (-243.6348, 86.5518) -> (-242.8648, 86.5518)
  arc A18 (-242.6148, 86.5414) -> (-242.8648, 86.5518) centre (-242.8648, 83.5518) ccw
  arc A19 (-242.3648, 86.5518) -> (-242.6148, 86.5414) centre (-242.3648, 83.5518) ccw
  line L94 (-242.3648, 86.5518) -> (-241.5148, 86.5518)
  arc A20 (-241.3048, 86.5445) -> (-241.5148, 86.5518) centre (-241.5148, 83.5518) ccw
  arc A21 (-241.0948, 86.5518) -> (-241.3048, 86.5445) centre (-241.0948, 83.5518) ccw
  line L95 (-241.0948, 86.5518) -> (-240.3248, 86.5518)
  arc A22 (-240.0748, 86.5414) -> (-240.3248, 86.5518) centre (-240.3248, 83.5518) ccw
  arc A23 (-239.8248, 86.5518) -> (-240.0748, 86.5414) centre (-239.8248, 83.5518) ccw
  line L96 (-239.8248, 86.5518) -> (-239.0548, 86.5518)
  arc A24 (-238.8048, 86.5414) -> (-239.0548, 86.5518) centre (-239.0548, 83.5518) ccw
  arc A25 (-238.5548, 86.5518) -> (-238.8048, 86.5414) centre (-238.5548, 83.5518) ccw
  line L97 (-238.5548, 86.5518) -> (-237.7848, 86.5518)
  arc A26 (-237.5348, 86.5414) -> (-237.7848, 86.5518) centre (-237.7848, 83.5518) ccw
  arc A27 (-237.2848, 86.5518) -> (-237.5348, 86.5414) centre (-237.2848, 83.5518) ccw
  line L98 (-237.2848, 86.5518) -> (-236.5148, 86.5518)
  arc A28 (-236.2648, 86.5414) -> (-236.5148, 86.5518) centre (-236.5148, 83.5518) ccw
  arc A29 (-236.0148, 86.5518) -> (-236.2648, 86.5414) centre (-236.0148, 83.5518) ccw
  line L99 (-236.0148, 86.5518) -> (-235.2448, 86.5518)
  arc A30 (-234.9948, 86.5414) -> (-235.2448, 86.5518) centre (-235.2448, 83.5518) ccw
  arc A31 (-234.7448, 86.5518) -> (-234.9948, 86.5414) centre (-234.7448, 83.5518) ccw
  line L100 (-234.7448, 86.5518) -> (-233.9748, 86.5518)
  arc A32 (-233.7248, 86.5414) -> (-233.9748, 86.5518) centre (-233.9748, 83.5518) ccw
  arc A33 (-233.4748, 86.5518) -> (-233.7248, 86.5414) centre (-233.4748, 83.5518) ccw
  line L101 (-233.4748, 86.5518) -> (-232.7048, 86.5518)
  arc A34 (-232.4548, 86.5414) -> (-232.7048, 86.5518) centre (-232.7048, 83.5518) ccw
  arc A35 (-232.2048, 86.5518) -> (-232.4548, 86.5414) centre (-232.2048, 83.5518) ccw
  line L102 (-232.2048, 86.5518) -> (-199.377, 86.5518)
  line L103 (-199.377, 86.5518) -> (-199.377, 118.6521)
  line L104 (-199.377, 118.6521) -> (-338.527, 118.6521)
  line L105 (-338.527, 118.6521) -> (-338.527, 36.7921)
  line L106 (-338.527, 36.7921) -> (-199.377, 36.7921)
  line L107 (-199.377, 36.7921) -> (-199.377, 62.5518)
  line L108 (-199.377, 62.5518) -> (-232.2048, 62.5518)
  arc A36 (-232.4548, 62.5622) -> (-232.2048, 62.5518) centre (-232.2048, 65.5518) ccw
  arc A37 (-232.7048, 62.5518) -> (-232.4548, 62.5622) centre (-232.7048, 65.5518) ccw
  line L109 (-232.7048, 62.5518) -> (-233.4748, 62.5518)
  arc A38 (-233.633, 62.556) -> (-233.4748, 62.5518) centre (-233.4748, 65.5518) ccw
  line L110 (-233.633, 62.556) -> (-233.633, 53)
  line L111 (-233.633, 53) -> (-245.633, 53)
  line L112 (-245.633, 53) -> (-245.633, 62.5518)
  line L113 (-245.633, 62.5518) -> (-246.1748, 62.5518)
  arc A39 (-246.4248, 62.5622) -> (-246.1748, 62.5518) centre (-246.1748, 65.5518) ccw
  arc A40 (-246.6748, 62.5518) -> (-246.4248, 62.5622) centre (-246.6748, 65.5518) ccw
  line L114 (-246.6748, 62.5518) -> (-247.4448, 62.5518)
  arc A41 (-247.6948, 62.5622) -> (-247.4448, 62.5518) centre (-247.4448, 65.5518) ccw
  arc A42 (-247.9448, 62.5518) -> (-247.6948, 62.5622) centre (-247.9448, 65.5518) ccw
  line L115 (-247.9448, 62.5518) -> (-248.7148, 62.5518)
  arc A43 (-248.9648, 62.5622) -> (-248.7148, 62.5518) centre (-248.7148, 65.5518) ccw
  arc A44 (-249.2148, 62.5518) -> (-248.9648, 62.5622) centre (-249.2148, 65.5518) ccw
  line L116 (-249.2148, 62.5518) -> (-252.4198, 62.5518)
  arc A45 (-253.4198, 63.5518) -> (-252.4198, 62.5518) centre (-252.4198, 63.5518) ccw
  line L117 (-253.4198, 63.5518) -> (-253.4198, 68.5418)
  arc A46 (-253.4094, 68.7918) -> (-253.4198, 68.5418) centre (-250.4198, 68.5418) ccw
  arc A47 (-253.4198, 69.0418) -> (-253.4094, 68.7918) centre (-250.4198, 69.0418) ccw
  line L118 (-253.4198, 69.0418) -> (-253.4198, 69.8118)
  arc A48 (-253.4094, 70.0618) -> (-253.4198, 69.8118) centre (-250.4198, 69.8118) ccw
  arc A49 (-253.4198, 70.3118) -> (-253.4094, 70.0618) centre (-250.4198, 70.3118) ccw
  line L119 (-253.4198, 70.3118) -> (-253.4198, 71.0818)
  arc A50 (-253.4094, 71.3318) -> (-253.4198, 71.0818) centre (-250.4198, 71.0818) ccw
  arc A51 (-253.4198, 71.5818) -> (-253.4094, 71.3318) centre (-250.4198, 71.5818) ccw
  line L120 (-253.4198, 71.5818) -> (-253.4198, 72.3518)
  arc A52 (-253.4094, 72.6018) -> (-253.4198, 72.3518) centre (-250.4198, 72.3518) ccw
  arc A53 (-253.4198, 72.8518) -> (-253.4094, 72.6018) centre (-250.4198, 72.8518) ccw
  line L121 (-253.4198, 72.8518) -> (-253.4198, 73.6218)
  arc A54 (-253.4094, 73.8718) -> (-253.4198, 73.6218) centre (-250.4198, 73.6218) ccw
  arc A55 (-253.4198, 74.1218) -> (-253.4094, 73.8718) centre (-250.4198, 74.1218) ccw
  line L122 (-253.4198, 74.1218) -> (-253.4198, 74.8918)
  arc A56 (-253.4094, 75.1418) -> (-253.4198, 74.8918) centre (-250.4198, 74.8918) ccw
  arc A57 (-253.4198, 75.3918) -> (-253.4094, 75.1418) centre (-250.4198, 75.3918) ccw
  line L123 (-253.4198, 75.3918) -> (-253.4198, 76.1618)
  arc A58 (-253.4094, 76.4118) -> (-253.4198, 76.1618) centre (-250.4198, 76.1618) ccw